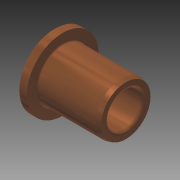
# Autodesk Inventor part: SHFZ12_25
Saved by Autodesk Inventor 2012 (Build 160160000, 160)
## iProperties
Category: PARTsolutions
Created: 2011-11-05
Part Number: SHFZ12_25
Catalog Web Link: www.cadenas.de
Description: SHFZ - Oil Free Bushings - Bronze, Flanged Type
Document SubType Name: Modeling
Designer: PARTsolutions
Material: Default
Density: 1 g/cm^3
NB: SHFZ12-25
NN: SHFZ
NT: Oil Free Bushings - Bronze, Flanged Type
NBSYN: $PN.
LINA: SHFZ12-25
PN: SHFZ12-25
MAT: Special Bronze Cast
HR: -40~150
DD: 12
DDTOL: +0.050/+0.032
L: 25
L1: 10,12,15,20,25,30
ALT11: '', 'w/o LC (Full Length)', '-LC', 'with LC (Full Length)'
LC: 0
LC1: [0]
LCMIN: 10
LCMAX: 24
D: 18
DTOL: +0.034/+0.023
T: 3
H: 25
TT: 3
TTTOL: 0/-0.1
HD: 18
HDTOL: +0.018/0
C: 0.400
R1: 0.400
R2: 1.000
LL: 1.500
KT: DUMMY
CreationOption_UseAsmMates: 0
SUPPLIER: Misumi
ARTICLENO: SHFZ12-25
BOMINFO: SHFZ12-25
CREATOR: CADENAS GmbH
PSOL_IDENT_0: {\\10.0.0.251\ps_data\23d-libs\misumi\metric\05_oil_free_bushings\shfz.prj},167 {VTYP=3D},{NB=SHFZ12
PSOL_IDENT_1: -25},{LINA=SHFZ12-25},{NN=SHFZ},{DATE=03.01.2011 06:59:00},{GEOMDATE=09.05.2008 00:00:00},{VERSION=}
PSOL_IDENT_2: ,{LINEID=50},{LINESUBID=-1},{WBVAR=L,ALT1,LC}  {NB=SHFZ12-25},{LINA=SHFZ12-25},{KT=DUMMY},{PN=SHFZ12
PSOL_IDENT_3: -25},{MAT=Special Bronze Cast},{HR=-40~150},{DD=12},{DDTOL=+0.050/+0.032},{L=25},{L1=10,12,15,20,25,
PSOL_IDENT_4: 30},{ALT1=},{ALT11= '', 'w/o LC (Full Length)', '-LC', 'with LC (Full Length)' },{LC=0},{LC1=[0]},{L
PSOL_IDENT_5: CMIN=10},{LCMAX=24},{D=18},{DTOL=+0.034/+0.023},{T=3},{H=25},{TT=3},{TTTOL=0/-0.1},{HD=18},{HDTOL=+0
PSOL_IDENT_6: .018/0},{C=0.400},{R1=0.400},{R2=1.000},{LL=1.500},{LCPN=}
Title: SHFZ12-25
Author: Cadenas PARTsolutions
Comments: Oil Free Bushings - Bronze, Flanged Type
Autodesk Inventor part; units mm, degrees
ref_plane "YZ Plane" through (0, 0, 0) normal (1, 0, 0) x (0, 1, 0)
ref_plane "XZ Plane" through (0, 0, 0) normal (0, 1, 0) x (-1, 0, 0)
ref_plane "XY Plane" through (0, 0, 0) normal (0, 0, 1) x (1, 0, 0)
sketch "Sketch_1" plane through (0, 0, 0) normal (0, 0, 1) x (1, 0, 0)
  line L0 (25, 0) -> (0, 0)
  line L1 (0, 12.1) -> (0, 7)
  arc A0 (0, 7) -> (1, 6) centre (1, 7) ccw
  line L2 (1, 6) -> (24, 6)
  arc A1 (24, 6) -> (25, 7) centre (24, 7) ccw
  line L3 (25, 7) -> (25, 8.5981)
  line L4 (25, 8.5981) -> (23.5, 9)
  line L5 (23.5, 9) -> (3.4, 9)
  arc A2 (3, 9.4) -> (3.4, 9) centre (3.4, 9.4) ccw
  line L6 (3, 9.4) -> (3, 12.5)
  line L7 (3, 12.5) -> (0.4, 12.5)
  line L8 (0.4, 12.5) -> (0, 12.1)
  constraints: 18 end point, 6 point on circle, 3 centre point
revolve "Revolution1" add sketch "Sketch_1" angle 360 about axis through (25, 0, 0) along (1, 0, 0)
body "Solid1"
